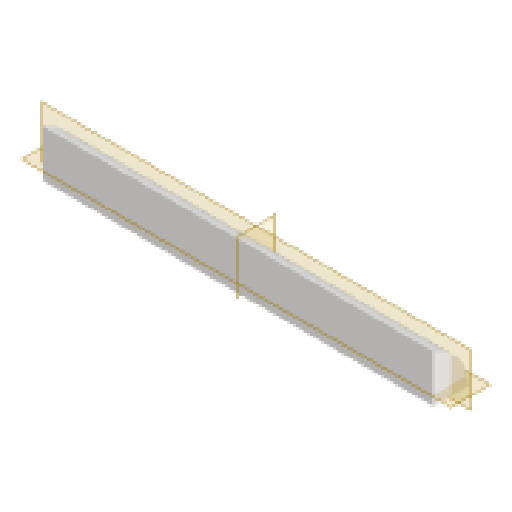
# Autodesk Inventor part: Край задней части корпуса
Saved by Autodesk Inventor 2023.2 (Build 272271030, 271C)
## iProperties
Created: 2025-04-24
Part Number: Край задней части корпуса
Material: Типовые
Document SubType Name: Modeling
Designer: Коноваленко
Density: 1 g/cm^3
Appearance: По умолчанию
Author: Коноваленко
Autodesk Inventor part; units mm, degrees
sketch "Эскиз1" plane through (0, 0, 0) normal (1, 0, 0) x (0, 1, 0)
  line L0 (-8.3221, -14.9171) -> (-8.3221, 15.0829)
  line L1 (-8.3221, 15.0829) -> (31.6779, 15.0829)
  arc A0 (-8.3221, -14.9171) -> (31.6779, 15.0829) centre (-10.7721, 30.0161) ccw
  point P0 (0, 0)
  dimension "d0" = 30
  dimension "d1" = 40
  dimension "d5" = 45
  constraints: 4 end point, 2 point on circle, 1 centre point, 1 horizontal, 1 vertical
  measures "d0" distance of L0.start L0.end
  measures "d1" distance of L0.end L1.end
  measures "d5" radius of A0
extrude "Выдавливание1" add sketch "Эскиз1" along normal mid plane 330
